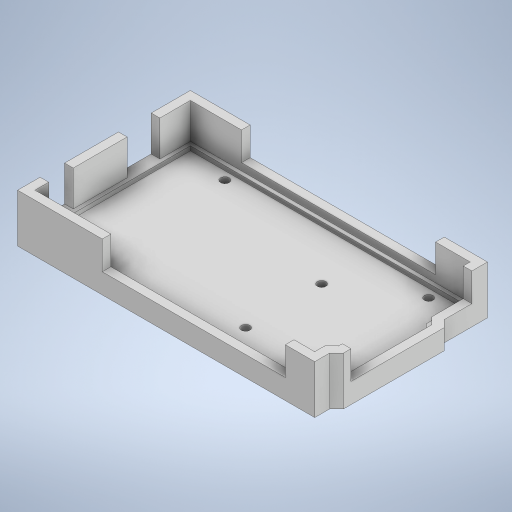
# Autodesk Inventor part: ArduinoMegaCaseBottom
Saved by Autodesk Inventor 2024 (Build 280153000, 153)
## iProperties
Created: 2023-07-08
Part Number: ArduinoMegaCaseBottom
Material: Generic
Document SubType Name: Modeling
Designer: 18179
Density: 1 g/cm^3
Appearance: Default
Author: 18179
Autodesk Inventor part; units mm, degrees
ref_plane "YZ Plane" through (0, 0, 0) normal (1, 0, 0) x (0, 1, 0)
ref_plane "XZ Plane" through (0, 0, 0) normal (0, 1, 0) x (-1, 0, 0)
ref_plane "XY Plane" through (0, 0, 0) normal (0, 0, 1) x (1, 0, 0)
sketch "Sketch1" plane through (0, 0, 0) normal (0, 1, 0) x (-1, 0, 0)
  line L0 (0, 0) -> (0, -53.34)
  line L1 (0, -53.34) -> (0, -50.165)
  line L2 (0, -50.165) -> (1.905, -50.165)
  line L3 (1.905, -50.165) -> (0, -50.165)
  line L4 (0, -50.165) -> (0, -41.165)
  line L5 (0, -41.165) -> (1.905, -41.165)
  line L6 (1.905, -41.165) -> (1.905, -50.165)
  line L7 (0, 0) -> (0, -9.3)
  line L8 (0, -9.3) -> (6.35, -9.3)
  line L9 (6.35, -9.3) -> (0, -9.3)
  line L10 (0, -9.3) -> (0, -21.34)
  line L11 (0, -21.34) -> (6.35, -21.34)
  line L12 (6.35, -21.34) -> (6.35, -9.3)
  line L13 (0, -53.34) -> (-99.06, -53.34)
  line L14 (0, 0) -> (-99.06, 0)
  line L15 (0, -53.34) -> (-13.67, -53.34) construction
  line L16 (-13.67, -53.34) -> (-13.67, -50.8) construction
  line L17 (-13.67, -50.8) -> (0, -50.8) construction
  line L18 (0, -50.8) -> (0, -53.34) construction
  line L19 (0, 0) -> (-15.24, 0) construction
  line L20 (-15.24, 0) -> (-15.24, -2.54) construction
  line L21 (-15.24, -2.54) -> (0, -2.54) construction
  line L22 (0, -2.54) -> (0, 0) construction
  line L23 (-99.06, 0) -> (-90.17, 0) construction
  line L24 (-90.17, 0) -> (-90.17, -2.54) construction
  line L25 (-90.17, -2.54) -> (-99.06, -2.54) construction
  line L26 (-99.06, -2.54) -> (-99.06, 0) construction
  line L27 (-99.06, -53.34) -> (-96.52, -53.34) construction
  line L28 (-96.52, -53.34) -> (-96.52, -50.8) construction
  line L29 (-96.52, -50.8) -> (-99.06, -50.8) construction
  line L30 (-99.06, -50.8) -> (-99.06, -53.34) construction
  line L31 (-99.06, 0) -> (-66.04, 0) construction
  line L32 (-66.04, 0) -> (-66.04, -17.78) construction
  line L33 (-66.04, -17.78) -> (-99.06, -17.78) construction
  line L34 (-99.06, -17.78) -> (-99.06, 0) construction
  line L35 (-99.06, -53.34) -> (-66.04, -53.34) construction
  line L36 (-66.04, -53.34) -> (-66.04, -45.72) construction
  line L37 (-66.04, -45.72) -> (-99.06, -45.72) construction
  line L38 (-99.06, -45.72) -> (-99.06, -53.34) construction
  line L39 (-99.06, 0) -> (-99.06, -12.954)
  line L40 (-99.06, -53.34) -> (-99.06, -50.8)
  line L41 (-99.06, -50.8) -> (-101.6, -50.8) construction
  line L42 (-101.6, -50.8) -> (-101.6, -48.26) construction
  line L43 (-101.6, -48.26) -> (-99.06, -48.26) construction
  line L44 (-99.06, -48.26) -> (-99.06, -50.8) construction
  line L45 (-99.06, -12.954) -> (-101.6, -12.954) construction
  line L46 (-101.6, -12.954) -> (-101.6, -15.494) construction
  line L47 (-101.6, -15.494) -> (-99.06, -15.494) construction
  line L48 (-99.06, -15.494) -> (-99.06, -12.954) construction
  line L49 (-99.06, -12.954) -> (-101.6, -15.494)
  line L50 (-101.6, -15.494) -> (-101.6, -48.26)
  line L51 (-101.6, -48.26) -> (-99.06, -50.8)
  circle A0 centre (-13.67, -50.8) radius 1.5875
  circle A1 centre (-15.24, -2.54) radius 1.5875
  circle A2 centre (-66.04, -17.78) radius 1.5875
  circle A3 centre (-66.04, -45.72) radius 1.5875
  circle A4 centre (-96.52, -50.8) radius 1.5875
  circle A5 centre (-90.17, -2.54) radius 1.5875
  line L52 (0, -58.42) -> (-104.14, -58.42)
  line L53 (-104.14, -58.42) -> (-104.14, -52.9042)
  line L54 (-104.14, -52.9042) -> (-106.68, -50.3642)
  line L55 (-106.68, -50.3642) -> (-106.68, -13.3898)
  line L56 (-106.68, -13.3898) -> (-104.14, -10.8498)
  line L57 (-104.14, -10.8498) -> (-104.14, 5.08)
  line L58 (-104.14, 5.08) -> (0, 5.08)
  line L59 (0, -55.245) -> (-100.965, -55.245)
  line L60 (-100.965, -55.245) -> (-100.965, -51.5891)
  line L61 (-100.965, -51.5891) -> (-103.505, -49.0491)
  line L62 (-103.505, -49.0491) -> (-103.505, -14.7049)
  line L63 (-103.505, -14.7049) -> (-100.965, -12.1649)
  line L64 (-100.965, -12.1649) -> (-100.965, 1.905)
  line L65 (-100.965, 1.905) -> (0, 1.905)
  line L66 (5.08, 0) -> (5.08, -53.34)
  line L67 (1.905, 0) -> (1.905, -53.34)
  line L68 (0, -58.42) -> (5.08, -58.42)
  line L69 (5.08, -58.42) -> (5.08, -53.34)
  line L70 (1.905, -53.34) -> (1.905, -55.245)
  line L71 (1.905, -55.245) -> (0, -55.245)
  line L72 (1.905, 0) -> (1.905, 1.905)
  line L73 (1.905, 1.905) -> (0, 1.905)
  line L74 (0, 5.08) -> (5.08, 5.08)
  line L75 (5.08, 5.08) -> (5.08, 0)
  dimension "d0" = 53.34
  dimension "d1" = 3.175
  dimension "d2" = 1.905
  dimension "d3" = 9
  dimension "d4" = 9.3
  dimension "d5" = 6.35
  dimension "d6" = 12.04
  dimension "d7" = 99.06
  dimension "d8" = 99.06
  dimension "d9" = 13.67
  dimension "d10" = 2.54
  dimension "d11" = 15.24
  dimension "d12" = 2.54
  dimension "d13" = 8.89
  dimension "d14" = 2.54
  dimension "d15" = 2.54
  dimension "d16" = 2.54
  dimension "d17" = 17.78
  dimension "d18" = 33.02
  dimension "d19" = 33.02
  dimension "d20" = 7.62
  dimension "d21" = 12.954
  dimension "d22" = 2.54
  dimension "d23" = 2.54
  dimension "d24" = 2.54
  dimension "d25" = 2.54
  dimension "d26" = 2.54
  dimension "d27" = 3.175
  dimension "d28" = 3.175
  dimension "d29" = 3.175
  dimension "d30" = 3.175
  dimension "d31" = 3.175
  dimension "d32" = 3.175
  dimension "d33" = 5.08
  dimension "d34" = 3.175
  dimension "d35" = 5.08
  dimension "d36" = 3.175
  constraints: 152 end point, 23 parallel, 15 perpendicular, 14 horizontal, 7 point on line, 6 centre point, 6 coincident, 2 vertical, 1 collinear, 12 other
  measures "d0" distance of L0.start L0.end
  measures "d1" distance of L0.end L1.end
  measures "d2" distance of L1.end L2.end
  measures "d3" distance of L3.end L4.end
  measures "d4" distance of L0.start L7.end
  measures "d5" distance of L7.end L8.end
  measures "d6" distance of L10.end L9.end
  measures "d7" distance of L0.end L13.end
  measures "d8" distance of L0.start L14.end
  measures "d9" distance of L16.end L17.end
  measures "d10" distance of L15.end L16.end
  measures "d11" distance of L21.end L20.end
  measures "d12" distance of L20.end L19.end
  measures "d13" distance of L24.end L25.end
  measures "d14" distance of L23.end L24.end
  measures "d15" distance of L29.end L28.end
  measures "d16" distance of L28.end L27.end
  measures "d17" distance of L31.end L32.end
  measures "d18" distance of L32.end L33.end
  measures "d19" distance of L37.end L36.end
  measures "d20" distance of L36.end L35.end
  measures "d21" distance of L14.end L39.end
  measures "d22" distance of L13.end L29.end
  measures "d23" distance of L42.end L43.end
  measures "d24" distance of L41.end L42.end
  measures "d25" distance of L47.end L46.end
  measures "d26" distance of L46.end L45.end
  measures "d27" diameter of A0
  measures "d28" diameter of A1
  measures "d29" diameter of A2
  measures "d30" diameter of A3
  measures "d31" diameter of A4
  measures "d32" diameter of A5
  measures "d33" distance between parallel lines of L13 L52
  measures "d34" distance between parallel lines of L52 L59
  measures "d35" distance between parallel lines of L0 L66
  measures "d36" distance between parallel lines of L66 L67
sketch "Sketch2" plane through (0, 0, 0) normal (0, 1, 0) x (-1, 0, 0)
  line L0 (0, 0) -> (0, -53.34)
  line L1 (0, -53.34) -> (0, -50.165)
  line L2 (0, -50.165) -> (1.905, -50.165)
  line L3 (1.905, -50.165) -> (0, -50.165)
  line L4 (0, -50.165) -> (0, -41.165)
  line L5 (0, -41.165) -> (1.905, -41.165)
  line L6 (1.905, -41.165) -> (1.905, -50.165)
  line L7 (0, 0) -> (0, -9.3)
  line L8 (0, -9.3) -> (6.35, -9.3)
  line L9 (6.35, -9.3) -> (0, -9.3)
  line L10 (0, -9.3) -> (0, -21.34)
  line L11 (0, -21.34) -> (6.35, -21.34)
  line L12 (6.35, -21.34) -> (6.35, -9.3)
  line L13 (0, -53.34) -> (-99.06, -53.34)
  line L14 (0, 0) -> (-99.06, 0)
  line L15 (0, -53.34) -> (-13.67, -53.34) construction
  line L16 (-13.67, -53.34) -> (-13.67, -50.8) construction
  line L17 (-13.67, -50.8) -> (0, -50.8) construction
  line L18 (0, -50.8) -> (0, -53.34) construction
  line L19 (0, 0) -> (-15.24, 0) construction
  line L20 (-15.24, 0) -> (-15.24, -2.54) construction
  line L21 (-15.24, -2.54) -> (0, -2.54) construction
  line L22 (0, -2.54) -> (0, 0) construction
  line L23 (-99.06, 0) -> (-90.17, 0) construction
  line L24 (-90.17, 0) -> (-90.17, -2.54) construction
  line L25 (-90.17, -2.54) -> (-99.06, -2.54) construction
  line L26 (-99.06, -2.54) -> (-99.06, 0) construction
  line L27 (-99.06, -53.34) -> (-96.52, -53.34) construction
  line L28 (-96.52, -53.34) -> (-96.52, -50.8) construction
  line L29 (-96.52, -50.8) -> (-99.06, -50.8) construction
  line L30 (-99.06, -50.8) -> (-99.06, -53.34) construction
  line L31 (-99.06, 0) -> (-66.04, 0) construction
  line L32 (-66.04, 0) -> (-66.04, -17.78) construction
  line L33 (-66.04, -17.78) -> (-99.06, -17.78) construction
  line L34 (-99.06, -17.78) -> (-99.06, 0) construction
  line L35 (-99.06, -53.34) -> (-66.04, -53.34) construction
  line L36 (-66.04, -53.34) -> (-66.04, -45.72) construction
  line L37 (-66.04, -45.72) -> (-99.06, -45.72) construction
  line L38 (-99.06, -45.72) -> (-99.06, -53.34) construction
  line L39 (-99.06, 0) -> (-99.06, -12.954)
  line L40 (-99.06, -53.34) -> (-99.06, -50.8)
  line L41 (-99.06, -50.8) -> (-101.6, -50.8) construction
  line L42 (-101.6, -50.8) -> (-101.6, -48.26) construction
  line L43 (-101.6, -48.26) -> (-99.06, -48.26) construction
  line L44 (-99.06, -48.26) -> (-99.06, -50.8) construction
  line L45 (-99.06, -12.954) -> (-101.6, -12.954) construction
  line L46 (-101.6, -12.954) -> (-101.6, -15.494) construction
  line L47 (-101.6, -15.494) -> (-99.06, -15.494) construction
  line L48 (-99.06, -15.494) -> (-99.06, -12.954) construction
  line L49 (-99.06, -12.954) -> (-101.6, -15.494)
  line L50 (-101.6, -15.494) -> (-101.6, -48.26)
  line L51 (-101.6, -48.26) -> (-99.06, -50.8)
  circle A0 centre (-13.67, -50.8) radius 1.5875
  circle A1 centre (-15.24, -2.54) radius 1.5875
  circle A2 centre (-66.04, -17.78) radius 1.5875
  circle A3 centre (-66.04, -45.72) radius 1.5875
  circle A4 centre (-96.52, -50.8) radius 1.5875
  circle A5 centre (-90.17, -2.54) radius 1.5875
  line L52 (0, -58.42) -> (-104.14, -58.42)
  line L53 (-104.14, -58.42) -> (-104.14, -52.9042)
  line L54 (-104.14, -52.9042) -> (-106.68, -50.3642)
  line L55 (-106.68, -50.3642) -> (-106.68, -13.3898)
  line L56 (-106.68, -13.3898) -> (-104.14, -10.8498)
  line L57 (-104.14, -10.8498) -> (-104.14, 5.08)
  line L58 (-104.14, 5.08) -> (0, 5.08)
  line L59 (0, -55.245) -> (-100.965, -55.245)
  line L60 (-100.965, -55.245) -> (-100.965, -51.5891)
  line L61 (-100.965, -51.5891) -> (-103.505, -49.0491)
  line L62 (-103.505, -49.0491) -> (-103.505, -14.7049)
  line L63 (-103.505, -14.7049) -> (-100.965, -12.1649)
  line L64 (-100.965, -12.1649) -> (-100.965, 1.905)
  line L65 (-100.965, 1.905) -> (0, 1.905)
  line L66 (5.08, 0) -> (5.08, -53.34)
  line L67 (1.905, 0) -> (1.905, -53.34)
  line L68 (0, -58.42) -> (5.08, -58.42)
  line L69 (5.08, -58.42) -> (5.08, -53.34)
  line L70 (1.905, -53.34) -> (1.905, -55.245)
  line L71 (1.905, -55.245) -> (0, -55.245)
  line L72 (1.905, 0) -> (1.905, 1.905)
  line L73 (1.905, 1.905) -> (0, 1.905)
  line L74 (0, 5.08) -> (5.08, 5.08)
  line L75 (5.08, 5.08) -> (5.08, 0)
  dimension "d37" = 53.34
  dimension "d38" = 3.175
  dimension "d39" = 1.905
  dimension "d40" = 9
  dimension "d41" = 9.3
  dimension "d42" = 6.35
  dimension "d43" = 12.04
  dimension "d44" = 99.06
  dimension "d45" = 99.06
  dimension "d46" = 13.67
  dimension "d47" = 2.54
  dimension "d48" = 15.24
  dimension "d49" = 2.54
  dimension "d50" = 8.89
  dimension "d51" = 2.54
  dimension "d52" = 2.54
  dimension "d53" = 2.54
  dimension "d54" = 17.78
  dimension "d55" = 33.02
  dimension "d56" = 33.02
  dimension "d57" = 7.62
  dimension "d58" = 12.954
  dimension "d59" = 2.54
  dimension "d60" = 2.54
  dimension "d61" = 2.54
  dimension "d62" = 2.54
  dimension "d63" = 2.54
  dimension "d64" = 3.175
  dimension "d65" = 3.175
  dimension "d66" = 3.175
  dimension "d67" = 3.175
  dimension "d68" = 3.175
  dimension "d69" = 3.175
  dimension "d70" = 5.08
  dimension "d71" = 3.175
  dimension "d72" = 5.08
  dimension "d73" = 3.175
  constraints: 152 end point, 23 parallel, 15 perpendicular, 14 horizontal, 7 point on line, 6 centre point, 6 coincident, 2 vertical, 1 collinear, 12 other
  measures "d37" distance of L0.start L0.end
  measures "d38" distance of L0.end L1.end
  measures "d39" distance of L1.end L2.end
  measures "d40" distance of L3.end L4.end
  measures "d41" distance of L0.start L7.end
  measures "d42" distance of L7.end L8.end
  measures "d43" distance of L10.end L9.end
  measures "d44" distance of L0.end L13.end
  measures "d45" distance of L0.start L14.end
  measures "d46" distance of L16.end L17.end
  measures "d47" distance of L15.end L16.end
  measures "d48" distance of L21.end L20.end
  measures "d49" distance of L20.end L19.end
  measures "d50" distance of L24.end L25.end
  measures "d51" distance of L23.end L24.end
  measures "d52" distance of L29.end L28.end
  measures "d53" distance of L28.end L27.end
  measures "d54" distance of L31.end L32.end
  measures "d55" distance of L32.end L33.end
  measures "d56" distance of L37.end L36.end
  measures "d57" distance of L36.end L35.end
  measures "d58" distance of L14.end L39.end
  measures "d59" distance of L13.end L29.end
  measures "d60" distance of L42.end L43.end
  measures "d61" distance of L41.end L42.end
  measures "d62" distance of L47.end L46.end
  measures "d63" distance of L46.end L45.end
  measures "d64" diameter of A0
  measures "d65" diameter of A1
  measures "d66" diameter of A2
  measures "d67" diameter of A3
  measures "d68" diameter of A4
  measures "d69" diameter of A5
  measures "d70" distance between parallel lines of L13 L52
  measures "d71" distance between parallel lines of L52 L59
  measures "d72" distance between parallel lines of L0 L66
  measures "d73" distance between parallel lines of L66 L67
sketch "Sketch3" plane through (0, 0, 0) normal (0, 1, 0) x (-1, 0, 0)
  line L0 (0, 0) -> (0, -53.34)
  line L1 (0, -53.34) -> (0, -50.165)
  line L2 (0, -50.165) -> (1.905, -50.165)
  line L3 (1.905, -50.165) -> (0, -50.165)
  line L4 (0, -50.165) -> (0, -41.165)
  line L5 (0, -41.165) -> (1.905, -41.165)
  line L6 (1.905, -41.165) -> (1.905, -50.165)
  line L7 (0, 0) -> (0, -9.3)
  line L8 (0, -9.3) -> (6.35, -9.3)
  line L9 (6.35, -9.3) -> (0, -9.3)
  line L10 (0, -9.3) -> (0, -21.34)
  line L11 (0, -21.34) -> (6.35, -21.34)
  line L12 (6.35, -21.34) -> (6.35, -9.3)
  line L13 (0, -53.34) -> (-99.06, -53.34)
  line L14 (0, 0) -> (-99.06, 0)
  line L15 (0, -53.34) -> (-13.67, -53.34) construction
  line L16 (-13.67, -53.34) -> (-13.67, -50.8) construction
  line L17 (-13.67, -50.8) -> (0, -50.8) construction
  line L18 (0, -50.8) -> (0, -53.34) construction
  line L19 (0, 0) -> (-15.24, 0) construction
  line L20 (-15.24, 0) -> (-15.24, -2.54) construction
  line L21 (-15.24, -2.54) -> (0, -2.54) construction
  line L22 (0, -2.54) -> (0, 0) construction
  line L23 (-99.06, 0) -> (-90.17, 0) construction
  line L24 (-90.17, 0) -> (-90.17, -2.54) construction
  line L25 (-90.17, -2.54) -> (-99.06, -2.54) construction
  line L26 (-99.06, -2.54) -> (-99.06, 0) construction
  line L27 (-99.06, -53.34) -> (-96.52, -53.34) construction
  line L28 (-96.52, -53.34) -> (-96.52, -50.8) construction
  line L29 (-96.52, -50.8) -> (-99.06, -50.8) construction
  line L30 (-99.06, -50.8) -> (-99.06, -53.34) construction
  line L31 (-99.06, 0) -> (-66.04, 0) construction
  line L32 (-66.04, 0) -> (-66.04, -17.78) construction
  line L33 (-66.04, -17.78) -> (-99.06, -17.78) construction
  line L34 (-99.06, -17.78) -> (-99.06, 0) construction
  line L35 (-99.06, -53.34) -> (-66.04, -53.34) construction
  line L36 (-66.04, -53.34) -> (-66.04, -45.72) construction
  line L37 (-66.04, -45.72) -> (-99.06, -45.72) construction
  line L38 (-99.06, -45.72) -> (-99.06, -53.34) construction
  line L39 (-99.06, 0) -> (-99.06, -12.954)
  line L40 (-99.06, -53.34) -> (-99.06, -50.8)
  line L41 (-99.06, -50.8) -> (-101.6, -50.8) construction
  line L42 (-101.6, -50.8) -> (-101.6, -48.26) construction
  line L43 (-101.6, -48.26) -> (-99.06, -48.26) construction
  line L44 (-99.06, -48.26) -> (-99.06, -50.8) construction
  line L45 (-99.06, -12.954) -> (-101.6, -12.954) construction
  line L46 (-101.6, -12.954) -> (-101.6, -15.494) construction
  line L47 (-101.6, -15.494) -> (-99.06, -15.494) construction
  line L48 (-99.06, -15.494) -> (-99.06, -12.954) construction
  line L49 (-99.06, -12.954) -> (-101.6, -15.494)
  line L50 (-101.6, -15.494) -> (-101.6, -48.26)
  line L51 (-101.6, -48.26) -> (-99.06, -50.8)
  circle A0 centre (-13.67, -50.8) radius 1.5875
  circle A1 centre (-15.24, -2.54) radius 1.5875
  circle A2 centre (-66.04, -17.78) radius 1.5875
  circle A3 centre (-66.04, -45.72) radius 1.5875
  circle A4 centre (-96.52, -50.8) radius 1.5875
  circle A5 centre (-90.17, -2.54) radius 1.5875
  line L52 (0, -58.42) -> (-104.14, -58.42)
  line L53 (-104.14, -58.42) -> (-104.14, -52.9042)
  line L54 (-104.14, -52.9042) -> (-106.68, -50.3642)
  line L55 (-106.68, -50.3642) -> (-106.68, -13.3898)
  line L56 (-106.68, -13.3898) -> (-104.14, -10.8498)
  line L57 (-104.14, -10.8498) -> (-104.14, 5.08)
  line L58 (-104.14, 5.08) -> (0, 5.08)
  line L59 (0, -55.245) -> (-100.965, -55.245)
  line L60 (-100.965, -55.245) -> (-100.965, -51.5891)
  line L61 (-100.965, -51.5891) -> (-103.505, -49.0491)
  line L62 (-103.505, -49.0491) -> (-103.505, -14.7049)
  line L63 (-103.505, -14.7049) -> (-100.965, -12.1649)
  line L64 (-100.965, -12.1649) -> (-100.965, 1.905)
  line L65 (-100.965, 1.905) -> (0, 1.905)
  line L66 (5.08, 0) -> (5.08, -53.34)
  line L67 (1.905, 0) -> (1.905, -53.34)
  line L68 (0, -58.42) -> (5.08, -58.42)
  line L69 (5.08, -58.42) -> (5.08, -53.34)
  line L70 (1.905, -53.34) -> (1.905, -55.245)
  line L71 (1.905, -55.245) -> (0, -55.245)
  line L72 (1.905, 0) -> (1.905, 1.905)
  line L73 (1.905, 1.905) -> (0, 1.905)
  line L74 (0, 5.08) -> (5.08, 5.08)
  line L75 (5.08, 5.08) -> (5.08, 0)
  point P0 (5.08, -21.34)
  point P1 (1.905, -21.34)
  point P2 (1.905, -9.3)
  point P3 (5.08, -9.3)
  dimension "d74" = 53.34
  dimension "d75" = 3.175
  dimension "d76" = 1.905
  dimension "d77" = 9
  dimension "d78" = 9.3
  dimension "d79" = 6.35
  dimension "d80" = 12.04
  dimension "d81" = 99.06
  dimension "d82" = 99.06
  dimension "d83" = 13.67
  dimension "d84" = 2.54
  dimension "d85" = 15.24
  dimension "d86" = 2.54
  dimension "d87" = 8.89
  dimension "d88" = 2.54
  dimension "d89" = 2.54
  dimension "d90" = 2.54
  dimension "d91" = 17.78
  dimension "d92" = 33.02
  dimension "d93" = 33.02
  dimension "d94" = 7.62
  dimension "d95" = 12.954
  dimension "d96" = 2.54
  dimension "d97" = 2.54
  dimension "d98" = 2.54
  dimension "d99" = 2.54
  dimension "d100" = 2.54
  dimension "d101" = 3.175
  dimension "d102" = 3.175
  dimension "d103" = 3.175
  dimension "d104" = 3.175
  dimension "d105" = 3.175
  dimension "d106" = 3.175
  dimension "d107" = 5.08
  dimension "d108" = 3.175
  dimension "d109" = 5.08
  dimension "d110" = 3.175
  constraints: 152 end point, 23 parallel, 15 perpendicular, 14 horizontal, 7 point on line, 6 centre point, 6 coincident, 2 vertical, 1 collinear, 12 other
  measures "d74" distance of L0.start L0.end
  measures "d75" distance of L0.end L1.end
  measures "d76" distance of L1.end L2.end
  measures "d77" distance of L3.end L4.end
  measures "d78" distance of L0.start L7.end
  measures "d79" distance of L7.end L8.end
  measures "d80" distance of L10.end L9.end
  measures "d81" distance of L0.end L13.end
  measures "d82" distance of L0.start L14.end
  measures "d83" distance of L16.end L17.end
  measures "d84" distance of L15.end L16.end
  measures "d85" distance of L21.end L20.end
  measures "d86" distance of L20.end L19.end
  measures "d87" distance of L24.end L25.end
  measures "d88" distance of L23.end L24.end
  measures "d89" distance of L29.end L28.end
  measures "d90" distance of L28.end L27.end
  measures "d91" distance of L31.end L32.end
  measures "d92" distance of L32.end L33.end
  measures "d93" distance of L37.end L36.end
  measures "d94" distance of L36.end L35.end
  measures "d95" distance of L14.end L39.end
  measures "d96" distance of L13.end L29.end
  measures "d97" distance of L42.end L43.end
  measures "d98" distance of L41.end L42.end
  measures "d99" distance of L47.end L46.end
  measures "d100" distance of L46.end L45.end
  measures "d101" diameter of A0
  measures "d102" diameter of A1
  measures "d103" diameter of A2
  measures "d104" diameter of A3
  measures "d105" diameter of A4
  measures "d106" diameter of A5
  measures "d107" distance between parallel lines of L13 L52
  measures "d108" distance between parallel lines of L52 L59
  measures "d109" distance between parallel lines of L0 L66
  measures "d110" distance between parallel lines of L66 L67
sketch "Sketch4" plane through (0, 0, 0) normal (0, 1, 0) x (-1, 0, 0)
  line L0 (0, 0) -> (0, -53.34)
  line L1 (0, -53.34) -> (0, -50.165)
  line L2 (0, -50.165) -> (1.905, -50.165)
  line L3 (1.905, -50.165) -> (0, -50.165)
  line L4 (0, -50.165) -> (0, -41.165)
  line L5 (0, -41.165) -> (1.905, -41.165)
  line L6 (1.905, -41.165) -> (1.905, -50.165)
  line L7 (0, 0) -> (0, -9.3)
  line L8 (0, -9.3) -> (6.35, -9.3)
  line L9 (6.35, -9.3) -> (0, -9.3)
  line L10 (0, -9.3) -> (0, -21.34)
  line L11 (0, -21.34) -> (6.35, -21.34)
  line L12 (6.35, -21.34) -> (6.35, -9.3)
  line L13 (0, -53.34) -> (-99.06, -53.34)
  line L14 (0, 0) -> (-99.06, 0)
  line L15 (0, -53.34) -> (-13.67, -53.34) construction
  line L16 (-13.67, -53.34) -> (-13.67, -50.8) construction
  line L17 (-13.67, -50.8) -> (0, -50.8) construction
  line L18 (0, -50.8) -> (0, -53.34) construction
  line L19 (0, 0) -> (-15.24, 0) construction
  line L20 (-15.24, 0) -> (-15.24, -2.54) construction
  line L21 (-15.24, -2.54) -> (0, -2.54) construction
  line L22 (0, -2.54) -> (0, 0) construction
  line L23 (-99.06, 0) -> (-90.17, 0) construction
  line L24 (-90.17, 0) -> (-90.17, -2.54) construction
  line L25 (-90.17, -2.54) -> (-99.06, -2.54) construction
  line L26 (-99.06, -2.54) -> (-99.06, 0) construction
  line L27 (-99.06, -53.34) -> (-96.52, -53.34) construction
  line L28 (-96.52, -53.34) -> (-96.52, -50.8) construction
  line L29 (-96.52, -50.8) -> (-99.06, -50.8) construction
  line L30 (-99.06, -50.8) -> (-99.06, -53.34) construction
  line L31 (-99.06, 0) -> (-66.04, 0) construction
  line L32 (-66.04, 0) -> (-66.04, -17.78) construction
  line L33 (-66.04, -17.78) -> (-99.06, -17.78) construction
  line L34 (-99.06, -17.78) -> (-99.06, 0) construction
  line L35 (-99.06, -53.34) -> (-66.04, -53.34) construction
  line L36 (-66.04, -53.34) -> (-66.04, -45.72) construction
  line L37 (-66.04, -45.72) -> (-99.06, -45.72) construction
  line L38 (-99.06, -45.72) -> (-99.06, -53.34) construction
  line L39 (-99.06, 0) -> (-99.06, -12.954)
  line L40 (-99.06, -53.34) -> (-99.06, -50.8)
  line L41 (-99.06, -50.8) -> (-101.6, -50.8) construction
  line L42 (-101.6, -50.8) -> (-101.6, -48.26) construction
  line L43 (-101.6, -48.26) -> (-99.06, -48.26) construction
  line L44 (-99.06, -48.26) -> (-99.06, -50.8) construction
  line L45 (-99.06, -12.954) -> (-101.6, -12.954) construction
  line L46 (-101.6, -12.954) -> (-101.6, -15.494) construction
  line L47 (-101.6, -15.494) -> (-99.06, -15.494) construction
  line L48 (-99.06, -15.494) -> (-99.06, -12.954) construction
  line L49 (-99.06, -12.954) -> (-101.6, -15.494)
  line L50 (-101.6, -15.494) -> (-101.6, -48.26)
  line L51 (-101.6, -48.26) -> (-99.06, -50.8)
  circle A0 centre (-13.67, -50.8) radius 1.5875
  circle A1 centre (-15.24, -2.54) radius 1.5875
  circle A2 centre (-66.04, -17.78) radius 1.5875
  circle A3 centre (-66.04, -45.72) radius 1.5875
  circle A4 centre (-96.52, -50.8) radius 1.5875
  circle A5 centre (-90.17, -2.54) radius 1.5875
  line L52 (0, -58.42) -> (-104.14, -58.42)
  line L53 (-104.14, -58.42) -> (-104.14, -52.9042)
  line L54 (-104.14, -52.9042) -> (-106.68, -50.3642)
  line L55 (-106.68, -50.3642) -> (-106.68, -13.3898)
  line L56 (-106.68, -13.3898) -> (-104.14, -10.8498)
  line L57 (-104.14, -10.8498) -> (-104.14, 5.08)
  line L58 (-104.14, 5.08) -> (0, 5.08)
  line L59 (0, -55.245) -> (-100.965, -55.245)
  line L60 (-100.965, -55.245) -> (-100.965, -51.5891)
  line L61 (-100.965, -51.5891) -> (-103.505, -49.0491)
  line L62 (-103.505, -49.0491) -> (-103.505, -14.7049)
  line L63 (-103.505, -14.7049) -> (-100.965, -12.1649)
  line L64 (-100.965, -12.1649) -> (-100.965, 1.905)
  line L65 (-100.965, 1.905) -> (0, 1.905)
  line L66 (5.08, 0) -> (5.08, -53.34)
  line L67 (1.905, 0) -> (1.905, -53.34)
  line L68 (0, -58.42) -> (5.08, -58.42)
  line L69 (5.08, -58.42) -> (5.08, -53.34)
  line L70 (1.905, -53.34) -> (1.905, -55.245)
  line L71 (1.905, -55.245) -> (0, -55.245)
  line L72 (1.905, 0) -> (1.905, 1.905)
  line L73 (1.905, 1.905) -> (0, 1.905)
  line L74 (0, 5.08) -> (5.08, 5.08)
  line L75 (5.08, 5.08) -> (5.08, 0)
  line L76 (-99.5516, -53.8316) -> (0.4916, -53.8316)
  line L77 (0.4916, -53.8316) -> (0.4916, -53.34)
  line L78 (0.4916, -53.34) -> (0.4916, 0)
  line L79 (0.4916, 0) -> (0.4916, 0.4916)
  line L80 (0.4916, 0.4916) -> (-99.5516, 0.4916)
  line L81 (-99.5516, 0.4916) -> (-99.5516, -12.7504)
  line L82 (-99.5516, -12.7504) -> (-102.0916, -15.2904)
  line L83 (-102.0916, -15.2904) -> (-102.0916, -48.4636)
  line L84 (-102.0916, -48.4636) -> (-99.5516, -51.0036)
  line L85 (-99.5516, -51.0036) -> (-99.5516, -53.8316)
  dimension "d111" = 53.34
  dimension "d112" = 3.175
  dimension "d113" = 1.905
  dimension "d114" = 9
  dimension "d115" = 9.3
  dimension "d116" = 6.35
  dimension "d117" = 12.04
  dimension "d118" = 99.06
  dimension "d119" = 99.06
  dimension "d120" = 13.67
  dimension "d121" = 2.54
  dimension "d122" = 15.24
  dimension "d123" = 2.54
  dimension "d124" = 8.89
  dimension "d125" = 2.54
  dimension "d126" = 2.54
  dimension "d127" = 2.54
  dimension "d128" = 17.78
  dimension "d129" = 33.02
  dimension "d130" = 33.02
  dimension "d131" = 7.62
  dimension "d132" = 12.954
  dimension "d133" = 2.54
  dimension "d134" = 2.54
  dimension "d135" = 2.54
  dimension "d136" = 2.54
  dimension "d137" = 2.54
  dimension "d138" = 3.175
  dimension "d139" = 3.175
  dimension "d140" = 3.175
  dimension "d141" = 3.175
  dimension "d142" = 3.175
  dimension "d143" = 3.175
  dimension "d144" = 5.08
  dimension "d145" = 3.175
  dimension "d146" = 5.08
  dimension "d147" = 3.175
  constraints: 172 end point, 23 parallel, 15 perpendicular, 14 horizontal, 7 point on line, 6 centre point, 6 coincident, 2 vertical, 1 collinear, 21 other
  measures "d111" distance of L0.start L0.end
  measures "d112" distance of L0.end L1.end
  measures "d113" distance of L1.end L2.end
  measures "d114" distance of L3.end L4.end
  measures "d115" distance of L0.start L7.end
  measures "d116" distance of L7.end L8.end
  measures "d117" distance of L10.end L9.end
  measures "d118" distance of L0.end L13.end
  measures "d119" distance of L0.start L14.end
  measures "d120" distance of L16.end L17.end
  measures "d121" distance of L15.end L16.end
  measures "d122" distance of L21.end L20.end
  measures "d123" distance of L20.end L19.end
  measures "d124" distance of L24.end L25.end
  measures "d125" distance of L23.end L24.end
  measures "d126" distance of L29.end L28.end
  measures "d127" distance of L28.end L27.end
  measures "d128" distance of L31.end L32.end
  measures "d129" distance of L32.end L33.end
  measures "d130" distance of L37.end L36.end
  measures "d131" distance of L36.end L35.end
  measures "d132" distance of L14.end L39.end
  measures "d133" distance of L13.end L29.end
  measures "d134" distance of L42.end L43.end
  measures "d135" distance of L41.end L42.end
  measures "d136" distance of L47.end L46.end
  measures "d137" distance of L46.end L45.end
  measures "d138" diameter of A0
  measures "d139" diameter of A1
  measures "d140" diameter of A2
  measures "d141" diameter of A3
  measures "d142" diameter of A4
  measures "d143" diameter of A5
  measures "d144" distance between parallel lines of L13 L52
  measures "d145" distance between parallel lines of L52 L59
  measures "d146" distance between parallel lines of L0 L66
  measures "d147" distance between parallel lines of L66 L67
sketch "Sketch5" plane through (0, 0, 0) normal (0, 1, 0) x (-1, 0, 0)
  line L0 (0, 0) -> (0, -53.34)
  line L1 (0, -53.34) -> (0, -50.165)
  line L2 (0, -50.165) -> (1.905, -50.165)
  line L3 (1.905, -50.165) -> (0, -50.165)
  line L4 (0, -50.165) -> (0, -41.165)
  line L5 (0, -41.165) -> (1.905, -41.165)
  line L6 (1.905, -41.165) -> (1.905, -50.165)
  line L7 (0, 0) -> (0, -9.3)
  line L8 (0, -9.3) -> (6.35, -9.3)
  line L9 (6.35, -9.3) -> (0, -9.3)
  line L10 (0, -9.3) -> (0, -21.34)
  line L11 (0, -21.34) -> (6.35, -21.34)
  line L12 (6.35, -21.34) -> (6.35, -9.3)
  line L13 (0, -53.34) -> (-99.06, -53.34)
  line L14 (0, 0) -> (-99.06, 0)
  line L15 (0, -53.34) -> (-13.67, -53.34) construction
  line L16 (-13.67, -53.34) -> (-13.67, -50.8) construction
  line L17 (-13.67, -50.8) -> (0, -50.8) construction
  line L18 (0, -50.8) -> (0, -53.34) construction
  line L19 (0, 0) -> (-15.24, 0) construction
  line L20 (-15.24, 0) -> (-15.24, -2.54) construction
  line L21 (-15.24, -2.54) -> (0, -2.54) construction
  line L22 (0, -2.54) -> (0, 0) construction
  line L23 (-99.06, 0) -> (-90.17, 0) construction
  line L24 (-90.17, 0) -> (-90.17, -2.54) construction
  line L25 (-90.17, -2.54) -> (-99.06, -2.54) construction
  line L26 (-99.06, -2.54) -> (-99.06, 0) construction
  line L27 (-99.06, -53.34) -> (-96.52, -53.34) construction
  line L28 (-96.52, -53.34) -> (-96.52, -50.8) construction
  line L29 (-96.52, -50.8) -> (-99.06, -50.8) construction
  line L30 (-99.06, -50.8) -> (-99.06, -53.34) construction
  line L31 (-99.06, 0) -> (-66.04, 0) construction
  line L32 (-66.04, 0) -> (-66.04, -17.78) construction
  line L33 (-66.04, -17.78) -> (-99.06, -17.78) construction
  line L34 (-99.06, -17.78) -> (-99.06, 0) construction
  line L35 (-99.06, -53.34) -> (-66.04, -53.34) construction
  line L36 (-66.04, -53.34) -> (-66.04, -45.72) construction
  line L37 (-66.04, -45.72) -> (-99.06, -45.72) construction
  line L38 (-99.06, -45.72) -> (-99.06, -53.34) construction
  line L39 (-99.06, 0) -> (-99.06, -12.954)
  line L40 (-99.06, -53.34) -> (-99.06, -50.8)
  line L41 (-99.06, -50.8) -> (-101.6, -50.8) construction
  line L42 (-101.6, -50.8) -> (-101.6, -48.26) construction
  line L43 (-101.6, -48.26) -> (-99.06, -48.26) construction
  line L44 (-99.06, -48.26) -> (-99.06, -50.8) construction
  line L45 (-99.06, -12.954) -> (-101.6, -12.954) construction
  line L46 (-101.6, -12.954) -> (-101.6, -15.494) construction
  line L47 (-101.6, -15.494) -> (-99.06, -15.494) construction
  line L48 (-99.06, -15.494) -> (-99.06, -12.954) construction
  line L49 (-99.06, -12.954) -> (-101.6, -15.494)
  line L50 (-101.6, -15.494) -> (-101.6, -48.26)
  line L51 (-101.6, -48.26) -> (-99.06, -50.8)
  circle A0 centre (-13.67, -50.8) radius 1.5875
  circle A1 centre (-15.24, -2.54) radius 1.5875
  circle A2 centre (-66.04, -17.78) radius 1.5875
  circle A3 centre (-66.04, -45.72) radius 1.5875
  circle A4 centre (-96.52, -50.8) radius 1.5875
  circle A5 centre (-90.17, -2.54) radius 1.5875
  line L52 (0, -58.42) -> (-104.14, -58.42)
  line L53 (-104.14, -58.42) -> (-104.14, -52.9042)
  line L54 (-104.14, -52.9042) -> (-106.68, -50.3642)
  line L55 (-106.68, -50.3642) -> (-106.68, -13.3898)
  line L56 (-106.68, -13.3898) -> (-104.14, -10.8498)
  line L57 (-104.14, -10.8498) -> (-104.14, 5.08)
  line L58 (-104.14, 5.08) -> (0, 5.08)
  line L59 (0, -55.245) -> (-100.965, -55.245)
  line L60 (-100.965, -55.245) -> (-100.965, -51.5891)
  line L61 (-100.965, -51.5891) -> (-103.505, -49.0491)
  line L62 (-103.505, -49.0491) -> (-103.505, -14.7049)
  line L63 (-103.505, -14.7049) -> (-100.965, -12.1649)
  line L64 (-100.965, -12.1649) -> (-100.965, 1.905)
  line L65 (-100.965, 1.905) -> (0, 1.905)
  line L66 (5.08, 0) -> (5.08, -53.34)
  line L67 (1.905, 0) -> (1.905, -53.34)
  line L68 (0, -58.42) -> (5.08, -58.42)
  line L69 (5.08, -58.42) -> (5.08, -53.34)
  line L70 (1.905, -53.34) -> (1.905, -55.245)
  line L71 (1.905, -55.245) -> (0, -55.245)
  line L72 (1.905, 0) -> (1.905, 1.905)
  line L73 (1.905, 1.905) -> (0, 1.905)
  line L74 (0, 5.08) -> (5.08, 5.08)
  line L75 (5.08, 5.08) -> (5.08, 0)
  dimension "d22" = 2.54
  dimension "d148" = 53.34
  dimension "d149" = 3.175
  dimension "d150" = 1.905
  dimension "d151" = 9
  dimension "d152" = 9.3
  dimension "d153" = 6.35
  dimension "d154" = 12.04
  dimension "d155" = 99.06
  dimension "d156" = 99.06
  dimension "d157" = 13.67
  dimension "d158" = 2.54
  dimension "d159" = 15.24
  dimension "d160" = 2.54
  dimension "d161" = 8.89
  dimension "d162" = 2.54
  dimension "d163" = 2.54
  dimension "d164" = 2.54
  dimension "d165" = 17.78
  dimension "d166" = 33.02
  dimension "d167" = 33.02
  dimension "d168" = 7.62
  dimension "d169" = 12.954
  dimension "d170" = 2.54
  dimension "d171" = 2.54
  dimension "d172" = 2.54
  dimension "d173" = 2.54
  dimension "d174" = 2.54
  dimension "d175" = 3.175
  dimension "d176" = 3.175
  dimension "d177" = 3.175
  dimension "d178" = 3.175
  dimension "d179" = 3.175
  dimension "d180" = 3.175
  dimension "d181" = 5.08
  dimension "d182" = 3.175
  dimension "d183" = 5.08
  dimension "d184" = 3.175
  constraints: 152 end point, 23 parallel, 15 perpendicular, 14 horizontal, 7 point on line, 6 centre point, 6 coincident, 2 vertical, 1 collinear, 12 other
  measures "d148" distance of L0.start L0.end
  measures "d149" distance of L0.end L1.end
  measures "d150" distance of L1.end L2.end
  measures "d151" distance of L3.end L4.end
  measures "d152" distance of L0.start L7.end
  measures "d153" distance of L7.end L8.end
  measures "d154" distance of L10.end L9.end
  measures "d155" distance of L0.end L13.end
  measures "d156" distance of L0.start L14.end
  measures "d157" distance of L16.end L17.end
  measures "d158" distance of L15.end L16.end
  measures "d159" distance of L21.end L20.end
  measures "d160" distance of L20.end L19.end
  measures "d161" distance of L24.end L25.end
  measures "d162" distance of L23.end L24.end
  measures "d163" distance of L29.end L28.end
  measures "d164" distance of L28.end L27.end
  measures "d165" distance of L31.end L32.end
  measures "d166" distance of L32.end L33.end
  measures "d167" distance of L37.end L36.end
  measures "d168" distance of L36.end L35.end
  measures "d169" distance of L14.end L39.end
  measures "d170" distance of L13.end L29.end
  measures "d171" distance of L42.end L43.end
  measures "d172" distance of L41.end L42.end
  measures "d173" distance of L47.end L46.end
  measures "d174" distance of L46.end L45.end
  measures "d175" diameter of A0
  measures "d176" diameter of A1
  measures "d177" diameter of A2
  measures "d178" diameter of A3
  measures "d179" diameter of A4
  measures "d180" diameter of A5
  measures "d181" distance between parallel lines of L13 L52
  measures "d182" distance between parallel lines of L52 L59
  measures "d183" distance between parallel lines of L0 L66
  measures "d184" distance between parallel lines of L66 L67
extrude "Extrusion1" add sketch "Sketch5" against normal blind 3.175 contours L14 L39 L49 L50 L51 L40 L13 L0 L2 L67 L70 L71 L59 L60 L61 L62 L63 L64 L65 L73 L72 L8 | L0 L13 L40 L51 L50 L49 L39 L14 | L8 L67 L11 L0 | L11 L67 L5 L0 | L67 L72 L73 L65 L64 L63 L62 L61 L60 L59 L71 L70 L6 L11 L66 L69 L68 L52 L53 L54 L55 L56 L57 L58 L74 L75 L8 | L8 L66 L11 L67 | L5 L6 L2 L0
extrude "Extrusion2" add sketch "Sketch4" along normal blind 1.5875 contours L78 L79 L80 L81 L82 L83 L84 L85 L76 L77 L2 L67 L70 L71 L59 L60 L61 L62 L63 L64 L65 L73 L72 L8 | L8 L67 L11 L78 | L11 L67 L5 L78 | L67 L72 L73 L65 L64 L63 L62 L61 L60 L59 L71 L70 L6 L11 L66 L69 L68 L52 L53 L54 L55 L56 L57 L58 L74 L75 L8 | L8 L66 L11 L67 | L5 L6 L2 L78
extrude "Extrusion3" add sketch "Sketch3" along normal blind 14.619 contours L67 L72 L73 L65 L64 L63 L62 L61 L60 L59 L71 L70 L6 L11 L66 L69 L68 L52 L53 L54 L55 L56 L57 L58 L74 L75 L8
sketch "Sketch6" plane through (0, 14.619, 0) normal (0, 1, 0) x (1, 0, 0)
  line L0 (0, 50.165) -> (-1.905, 50.165) projected
  line L1 (0, 50.165) -> (0, 41.165) projected
  line L2 (0, 41.165) -> (-1.905, 41.165) projected
  line L3 (0, 50.165) -> (-7.8151, 50.165)
  line L4 (-7.8151, 50.165) -> (-7.8151, 41.165)
  line L5 (-7.8151, 41.165) -> (0, 41.165)
  line L6 (0, 41.165) -> (0, 50.165)
  point P0 (0, 0)
  constraints: 8 end point, 2 parallel, 1 horizontal, 1 perpendicular
extrude "Extrusion4" cut sketch "Sketch6" against normal up to surface (13.0315 mm away)
mirror "Mirror1" about plane through (104.14, 0, 5.08) normal (0, 0, 1) remove original yes
sketch "Sketch7" plane through (-5.08, 14.619, 68.58) normal (0, 1, 0) x (1, 0, 0)
  line L0 (0, 0) -> (109.22, 0) projected
  line L1 (0, 0) -> (31.115, 0)
  line L2 (3.175, 3.175) -> (106.045, 3.175) projected
  line L3 (31.115, 0) -> (98.425, 0)
  line L4 (98.425, 0) -> (98.425, 3.175)
  line L5 (98.425, 3.175) -> (31.115, 3.175)
  line L6 (31.115, 3.175) -> (31.115, 0)
  line L7 (0, 49.12) -> (0, 63.5) projected
  line L8 (0, 63.5) -> (21.971, 63.5)
  line L9 (0, 63.5) -> (109.22, 63.5) projected
  line L10 (106.045, 60.325) -> (3.175, 60.325) projected
  line L11 (21.971, 63.5) -> (93.345, 63.5)
  line L12 (93.345, 63.5) -> (93.345, 60.325)
  line L13 (93.345, 60.325) -> (21.971, 60.325)
  line L14 (21.971, 60.325) -> (21.971, 63.5)
  line L15 (109.22, 63.5) -> (109.22, 57.785)
  line L16 (109.22, 63.5) -> (109.22, 47.5702) projected
  line L17 (109.22, 57.785) -> (109.22, 10.795)
  line L18 (109.22, 10.795) -> (102.387, 10.795)
  line L19 (102.387, 10.795) -> (102.387, 57.785)
  line L20 (102.387, 57.785) -> (109.22, 57.785)
  line L21 (109.22, 57.785) -> (109.22, 10.795)
  line L22 (109.22, 10.795) -> (130.4223, 10.795)
  line L23 (130.4223, 10.795) -> (130.4223, 57.785)
  line L24 (130.4223, 57.785) -> (109.22, 57.785)
  line L25 (109.22, 57.785) -> (109.22, 10.795)
  point P0 (5.08, 68.58)
  point P1 (31.115, 3.175)
  point P2 (21.971, 60.325)
  dimension "d193" = 31.115
  dimension "d194" = 67.31
  dimension "d195" = 21.971
  dimension "d196" = 71.374
  dimension "d197" = 5.715
  dimension "d198" = 46.99
  constraints: 40 end point, 8 parallel, 7 point on line, 4 horizontal, 4 perpendicular
  measures "d193" distance of L0.start L1.end
  measures "d194" distance of L5.end L4.end
  measures "d195" distance of L7.end L8.end
  measures "d196" distance of L12.end L13.end
  measures "d197" distance of L9.end L15.end
  measures "d198" distance of L15.end L17.end
extrude "Extrusion5" cut sketch "Sketch7" against normal blind 10.414
body "Solid1"
